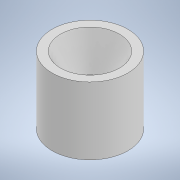
# Autodesk Inventor part: pierdolnik
Saved by Autodesk Inventor 2020 (Build 240168000, 168)
## iProperties
Created: 2019-12-28
Part Number: pierdolnik
Material: Ogólny
Document SubType Name: Modeling
Designer: macie
Density: 1 g/cm^3
Appearance: Domyślna
Author: macie
## iProperties of the stored document _Drukowanie 3D.ipt
Created: 2019-12-29
Part Number: _Drukowanie 3D
Material: Ogólny
Document SubType Name: Modeling
Designer: macie
Density: 1 g/cm^3
Appearance: Domyślna
Author: macie
Autodesk Inventor part; units mm, degrees
ref_plane "YZ Plane" through (0, 0, 0) normal (1, 0, 0) x (0, 1, 0)
ref_plane "XZ Plane" through (0, 0, 0) normal (0, 1, 0) x (-1, 0, 0)
ref_plane "XY Plane" through (0, 0, 0) normal (0, 0, 1) x (1, 0, 0)
sketch "Szkic1" plane through (0, 0, 0) normal (0, 0, 1) x (1, 0, 0)
  line L0 (0, 0) -> (1.5, 0) construction
  line L1 (0, 0) -> (4.5, 0) construction
  line L2 (4.5, 0) -> (4.5, 3.5)
  line L3 (0, 3.5) -> (3.5, 3.5) construction
  line L4 (4.5, 3.5) -> (3.5, 3.5)
  line L5 (3.5, 3.5) -> (1.5, 0)
  line L6 (1.5, 0) -> (4.5, 0)
  line L7 (0, 0) -> (0, 6.7021)
  dimension "d0" = 1.5
  dimension "d1" = 4.5
  dimension "d2" = 3.5
  dimension "d3" = 3.5
  constraints: 16 end point, 4 horizontal, 2 vertical, 1 collinear
  measures "d0" distance of L0.start L0.end
  measures "d1" distance of L0.start L1.end
  measures "d2" distance of L1.end L2.end
  measures "d3" distance of L3.start L3.end
revolve "Obrót1" add sketch "Szkic1" angle 360 about axis through (0, 0, 0) along (0, 1, 0)
sketch "Szkic2" plane through (0, 0, 0) normal (0, -1, 0) x (1, 0, 0)
  circle A0 centre (0, 0) radius 3.5 projected
  circle A1 centre (0, 0) radius 4.5 projected
  circle A2 centre (0, 0) radius 1.5 projected
extrude "Wyciągnięcie proste1" add sketch "Szkic2" along normal blind 4.5 contours A0 | A1
